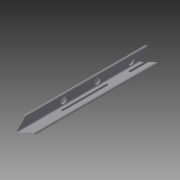
# Autodesk Inventor part: 2x2 quarter in angle aluminum number 2
Saved by Autodesk Inventor 2015 (Build 190159000, 159)
## iProperties
Created: 2015-02-01
Part Number: 2x2 quarter in angle aluminum number 2
Material: Generic
Document SubType Name: Modeling
Designer: szymsea16
Density: 1 g/cm^3
Appearance: Default
Author: szymsea16
Autodesk Inventor part; units mm, degrees
ref_plane "YZ Plane" through (0, 0, 0) normal (1, 0, 0) x (0, 1, 0)
ref_plane "XZ Plane" through (0, 0, 0) normal (0, 1, 0) x (-1, 0, 0)
ref_plane "XY Plane" through (0, 0, 0) normal (0, 0, 1) x (1, 0, 0)
sketch "Sketch1" plane through (0, 0, 0) normal (0, 1, 0) x (-1, 0, 0)
  line L0 (0, 0) -> (50.8, 0)
  line L1 (50.8, 0) -> (50.8, -736.6)
  line L2 (50.8, -736.6) -> (0, -736.6)
  line L3 (0, -736.6) -> (0, 0)
  dimension "d0" = 50.8
  dimension "d1" = 736.6
  constraints: 8 end point, 2 horizontal, 1 parallel, 1 perpendicular
  measures "d0" distance of L0.start L0.end
  measures "d1" distance of L0.end L1.end
extrude "Extrusion1" add sketch "Sketch1" along normal blind 6.35
sketch "Sketch2" plane through (0, 6.35, 0) normal (0, 1, 0) x (1, 0, 0)
  line L0 (-50.8, 0) -> (-44.45, 0)
  line L1 (-50.8, 0) -> (0, 0) projected
  line L2 (-44.45, 0) -> (-44.45, 736.6)
  line L3 (0, 736.6) -> (-50.8, 736.6) projected
  line L4 (-44.45, 736.6) -> (-50.8, 736.6)
  line L5 (-50.8, 736.6) -> (-50.8, 0)
  line L6 (-50.8, 0) -> (-44.45, 0)
  dimension "d4" = 6.35
  dimension "d5" = 736.6
  dimension "d6" = 736.6
  constraints: 10 end point, 1 perpendicular, 1 point on line, 1 vertical
  measures "d4" distance of L0.start L0.end
  measures "d5" distance of L0.end L2.end
  measures "d6" distance of L3.end L0.start
extrude "Extrusion2" add sketch "Sketch2" along normal blind 44.45
fillet "Fillet1" radius 6.35 1 edges at (-44.45, 6.35, -368.3)
fillet "Fillet2" radius 6.35 1 edges at (0, 6.35, -368.3)
fillet "Fillet3" radius 6.35 1 edges at (-44.45, 50.8, -368.3)
hole "Hole1" at (-44.45, 25.4, -247.65) direction (-1, 0, 0) diameter 28.575 end through all
pattern_linear "Rectangular Pattern1" count 3 spacing 152.4 along (0, 0, -1) of "Hole1"
hole "Hole2" at (-44.45, 28.575, -632.1298) direction (-1, 0, 0) diameter 15.24 end through all
sketch "Sketch4" plane through (0, 6.35, 0) normal (0, 1, 0) x (1, 0, 0)
  line L0 (-6.35, 736.6) -> (-6.35, 0) projected
  line L1 (-6.35, 736.6) -> (-38.1, 736.6) projected
  line L2 (-38.1, 0) -> (-38.1, 736.6) projected
  line L3 (-38.1, 0) -> (-6.35, 0) projected
  line L4 (0, 736.6) -> (0, 0) projected
  line L5 (-50.8, 736.6) -> (-50.8, 0) projected
  line L6 (-38.1, 0) -> (-38.1, 736.6) projected
  line L7 (-38.1, 703.0986) -> (0, 703.0986)
  line L8 (0, 703.0986) -> (0, 221.796)
  line L9 (0, 221.796) -> (-38.1, 221.796)
  line L10 (-38.1, 221.796) -> (-38.1, 703.0986)
  line L11 (-38.1, 221.796) -> (0, 200.8397)
  line L12 (0, 221.796) -> (-38.1, 221.796)
  line L13 (0, 221.796) -> (0, 200.8397)
  constraints: 14 end point, 3 point on line, 2 collinear, 2 parallel, 1 horizontal, 1 perpendicular
extrude "Extrusion3" cut sketch "Sketch4" against normal blind 25.4 contours L7 L4 L9 L0 | L0 L9 L2 L7 | L9 L4 L11 L0 | L0 L11 L9
sketch "Sketch7" plane through (-50.8, 0, -736.6) normal (-1, 0, 0) x (0, 0, 1)
  line L0 (736.6, 0) -> (736.6, 50.8) projected
  line L1 (736.6, 19.05) -> (658.9663, 96.6837)
  line L2 (736.6, 19.05) -> (846.3906, 19.05) construction
  line L3 (658.9663, 96.6837) -> (839.9542, 96.6837)
  line L4 (839.9542, 96.6837) -> (736.6, 19.05)
  dimension "d37" = 135
  constraints: 8 end point, 1 equal length, 1 horizontal, 1 perpendicular, 1 point on line
  measures "d37" angle of L2 L1
extrude "Extrusion4" cut sketch "Sketch7" against normal blind 25.4
sketch "Sketch8" plane through (-44.45, 12.7, 0) normal (1, 0, 0) x (0, 0, -1)
  line L0 (693.0898, 15.875) -> (693.0898, 61.5765)
  line L1 (693.0898, 61.5765) -> (693.0898, -44.6124)
  line L2 (693.0898, -44.6124) -> (800.4585, -39.8743)
  line L3 (800.4585, -39.8743) -> (791.1289, 38.6781)
  line L4 (791.1289, 38.6781) -> (744.7163, 67.7082)
  line L5 (744.7163, 67.7082) -> (693.0898, 61.5765)
  point P0 (0, -12.7)
  constraints: 12 end point, 1 perpendicular, 1 point on line
extrude "Extrusion5" cut sketch "Sketch8" along normal mid plane 96.8375
sketch "Sketch9" plane through (-50.8, 0, 0) normal (-1, 0, 0) x (0, 0, 1)
  line L0 (0, 0) -> (0, 6.35)
  line L1 (0, 6.35) -> (-221.796, 6.35) projected
  line L2 (-31.75, 50.8) -> (-57.15, 50.8)
  line L3 (-693.0898, 50.8) -> (-31.75, 50.8) projected
  line L4 (-57.15, 50.8) -> (0, 6.35)
  line L5 (37.7088, 23.9935) -> (15.7268, 85.5344)
  line L6 (15.7268, 85.5344) -> (-31.75, 88.3696)
  line L7 (-31.75, 88.3696) -> (-57.15, 50.8)
  line L8 (37.7088, 23.9935) -> (0, 6.35)
  dimension "d43" = 6.35
  dimension "d44" = 25.4
  constraints: 14 end point, 1 perpendicular, 1 point on line
  measures "d43" distance of L0.start L0.end
  measures "d44" distance of L2.start L2.end
extrude "Extrusion6" cut sketch "Sketch9" against normal blind 96.8375
sketch "Sketch10" plane through (-50.8, 0, -693.0898) normal (-1, 0, 0) x (0, 0, 1)
  line L0 (693.0898, 6.35) -> (635.9398, 50.8) projected
  line L1 (0, 50.8) -> (635.9398, 50.8) projected
  line L2 (0, 50.8) -> (0, 0) projected
  line L3 (693.0898, 0) -> (0, 0) projected
  line L4 (693.0898, 0) -> (693.0898, 6.35) projected
  circle A0 centre (60.96, 28.575) radius 7.62 projected
  circle A1 centre (140.6398, 25.4) radius 14.2875 projected
  circle A2 centre (293.0398, 25.4) radius 14.2875 projected
  circle A3 centre (445.4398, 25.4) radius 14.2875 projected
extrude "Extrusion7" cut sketch "Sketch10" against normal blind 685.8 contours A1 | A2 | A3
sketch "Sketch11" plane through (-50.8, 0, 0) normal (0, 0, 1) x (1, 0, 0)
  line L0 (12.7, 6.35) -> (0, 6.35) projected
  line L1 (0, 0) -> (0, 6.35) projected
  line L2 (50.8, 0) -> (0, 0) projected
  arc A0 (50.8, 0) -> (44.45, 6.35) centre (44.45, 0) ccw projected
  line L3 (12.7, 6.35) -> (44.45, 6.35) projected
extrude "Extrusion8" add sketch "Sketch11" against normal blind 693.039
sketch "Sketch12" plane through (0, 6.35, 0) normal (0, 1, 0) x (1, 0, 0)
  line L0 (-27.2437, 527.4945) -> (-27.2437, 577.4055) projected
  line L1 (-26.3547, 577.4055) -> (-26.3547, 527.4945) projected
  line L2 (-28.7677, 575.8815) -> (-28.7677, 529.0185) projected
  line L3 (-24.8307, 529.0185) -> (-24.8307, 575.8815) projected
  line L4 (-28.7677, 655.5613) -> (-28.7677, 608.6983) projected
  line L5 (-27.2437, 607.1743) -> (-27.2437, 657.0853) projected
  line L6 (-26.3547, 657.0853) -> (-26.3547, 607.1743) projected
  line L7 (-24.8307, 608.6983) -> (-24.8307, 655.5613) projected
  line L8 (-28.7677, 423.4815) -> (-28.7677, 376.6185) projected
  line L9 (-27.2437, 375.0945) -> (-27.2437, 425.0055) projected
  line L10 (-26.3547, 425.0055) -> (-26.3547, 375.0945) projected
  line L11 (-24.8307, 376.6185) -> (-24.8307, 423.4815) projected
  line L12 (-28.7677, 271.0815) -> (-28.7677, 224.2185) projected
  line L13 (-27.2437, 222.6945) -> (-27.2437, 272.6055) projected
  line L14 (-26.3547, 272.6055) -> (-26.3547, 222.6945) projected
  line L15 (-24.8307, 224.2185) -> (-24.8307, 271.0815) projected
  line L16 (-28.7677, 655.5613) -> (-24.8307, 655.5613)
  circle A0 centre (-26.7992, 655.5613) radius 4.7625
  line L17 (-28.7677, 529.0185) -> (-24.8307, 529.0185)
  circle A1 centre (-26.7992, 529.0185) radius 4.7625
  line L18 (-31.5617, 655.5613) -> (-22.0367, 655.5613)
  line L19 (-22.0367, 655.5613) -> (-22.0367, 529.0185)
  line L20 (-22.0367, 529.0185) -> (-31.5617, 529.0185)
  line L21 (-31.5617, 529.0185) -> (-31.5617, 655.5613)
  line L22 (-28.7677, 423.4815) -> (-24.8307, 423.4815)
  circle A2 centre (-26.7992, 423.4815) radius 4.7625
  line L23 (-28.7677, 224.2185) -> (-24.8307, 224.2185)
  circle A3 centre (-26.7992, 224.2185) radius 4.7625
  line L24 (-31.5617, 423.4815) -> (-22.0367, 423.4815)
  line L25 (-22.0367, 423.4815) -> (-22.0367, 224.2185)
  line L26 (-22.0367, 224.2185) -> (-31.5617, 224.2185)
  line L27 (-31.5617, 224.2185) -> (-31.5617, 423.4815)
  point P0 (0, 0)
  dimension "d51" = 9.525
  dimension "d52" = 9.525
  dimension "d53" = 9.525
  dimension "d54" = 9.525
  constraints: 24 end point, 5 horizontal, 4 horizontal alignment, 4 midpoint, 4 parallel, 3 perpendicular, 8 other
extrude "Extrusion9" cut sketch "Sketch12" against normal blind 693.039
sketch "Sketch13" plane through (0, 0, 0) normal (0, -1, 0) x (1, 0, 0)
  circle A0 centre (-10.8427, -11.176) radius 2.667 projected
  circle A1 centre (-33.7027, -8.89) radius 2.667 projected
  circle A2 centre (12.3983, -8.89) radius 2.667 projected
  line L0 (21.2883, -16.891) -> (-42.5927, -16.891) projected
  line L1 (21.2883, 7.747) -> (21.2883, -16.891) projected
  line L2 (9.8583, 7.747) -> (21.2883, 7.747) projected
  line L3 (9.8583, 0) -> (9.8583, 7.747) projected
  line L4 (-31.1627, 0) -> (9.8583, 0) projected
  line L5 (-31.1627, 7.747) -> (-31.1627, 0) projected
  line L6 (-42.5927, 7.747) -> (-31.1627, 7.747) projected
  line L7 (-42.5927, -16.891) -> (-42.5927, 7.747) projected
  point P0 (0, 0)
extrude "Extrusion10" cut sketch "Sketch13" against normal blind 693.039 contours A0 | A1
sketch "Sketch14" plane through (-44.45, 25.4, -247.65) normal (1, 0, 0) x (0, 0, -1)
  line L0 (360.7916, 16.353) -> (428.7482, 16.353)
  line L1 (428.7482, 16.353) -> (428.7482, -10.4265)
  line L2 (428.7482, -10.4265) -> (360.7916, -10.4265)
  line L3 (360.7916, -10.4265) -> (360.7916, 16.353)
  point P0 (-247.65, -25.4)
  constraints: 8 end point, 2 parallel, 1 horizontal, 1 perpendicular
extrude "Extrusion11" add sketch "Sketch14" against normal blind 6.35
sketch "Sketch15" plane through (-44.45, 25.4, -247.65) normal (1, 0, 0) x (0, 0, -1)
  circle A0 centre (384.4798, -5.08) radius 7.62 projected
  circle A1 centre (384.4798, -5.08) radius 9.525
  point P0 (-247.65, -25.4)
  dimension "d61" = 19.05
  constraints: 1 centre point, 1 coincident
  measures "d61" diameter of A1
extrude "Extrusion12" cut sketch "Sketch15" against normal blind 6.35 contours A0 | A1
sketch "Sketch16" plane through (-44.45, 25.4, -247.65) normal (-1, 0, 0) x (0, 0, 1)
  circle A0 centre (-384.4798, -5.08) radius 9.525 projected
  point P0 (247.65, -25.4)
extrude "Extrusion13" cut sketch "Sketch16" against normal blind 6.35
body "Solid1"
